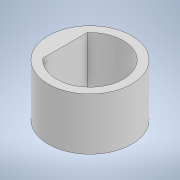
# Autodesk Inventor part: Prueba
Saved by Autodesk Inventor 2021 (Build 250183000, 183)
## iProperties
Created: 2022-04-27
Part Number: Prueba
Material: Genérico
Document SubType Name: Modeling
Designer: skatl
Density: 1 g/cm^3
Appearance: Valor por defecto
Author: skatl
Autodesk Inventor part; units mm, degrees
ref_plane "YZ Plane" through (0, 0, 0) normal (1, 0, 0) x (0, 1, 0)
ref_plane "XZ Plane" through (0, 0, 0) normal (0, 1, 0) x (-1, 0, 0)
ref_plane "XY Plane" through (0, 0, 0) normal (0, 0, 1) x (1, 0, 0)
sketch "Boceto1" plane through (0, 0, 0) normal (0, 1, 0) x (-1, 0, 0)
  circle A0 centre (0, 0) radius 3.2
  circle A1 centre (0, 0) radius 4
  line L0 (-3.2, 0) -> (2.4, 0)
  line L1 (2.4, 0) -> (2.4, -4.5231)
  line L2 (2.4, -4.5231) -> (2.4, 4.5638)
  point P0 (2.4, -2.1166)
  point P1 (2.4, 2.1166)
  dimension "d0" = 6.4
  dimension "d1" = 8
  dimension "d2" = 5.6
  constraints: 6 end point, 2 coincident, 1 centre point, 1 horizontal, 1 perpendicular, 1 point on line, 3 other
  measures "d1" diameter of A1
  measures "d2" distance of L0.start L0.end
extrude "Extrusión1" add sketch "Boceto1" along normal blind 5 contours A0 L1 L2 | A0 L2 A1 L1 | A0 L1 A1 L2
